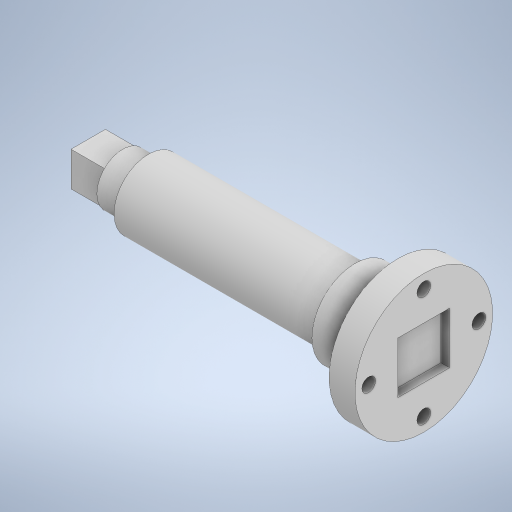
# Autodesk Inventor part: DRIVE SHAFT
Saved by Autodesk Inventor 2023 (Build 270158030, 158C)
## iProperties
Created: 2022-11-22
Part Number: DRIVE SHAFT
Material: Generic
Document SubType Name: Modeling
Designer: Imogen Heard
Density: 1 g/cm^3
Appearance: Default
Author: Imogen Heard
Autodesk Inventor part; units mm, degrees
ref_plane "YZ Plane" through (0, 0, 0) normal (1, 0, 0) x (0, 1, 0)
ref_plane "XZ Plane" through (0, 0, 0) normal (0, 1, 0) x (-1, 0, 0)
ref_plane "XY Plane" through (0, 0, 0) normal (0, 0, 1) x (1, 0, 0)
sketch "Sketch1" plane through (0, 0, 0) normal (1, 0, 0) x (0, 1, 0)
  circle A0 centre (0, 0) radius 40
  dimension "d0" = 80
  constraints: 1 centre point, 1 coincident
  measures "d0" diameter of A0
extrude "Extrusion1" add sketch "Sketch1" along normal blind 15
sketch "Sketch2" plane through (0, 0, 0) normal (-1, 0, 0) x (0, 0, 1)
  circle A0 centre (0, 0) radius 25
  circle A1 centre (0, 0) radius 40 projected
  dimension "d3" = 50
  constraints: 1 centre point, 1 concentric
  measures "d3" diameter of A0
extrude "Extrusion2" add sketch "Sketch2" along normal blind 25 contours A0
sketch "Sketch3" plane through (-25, 0, 0) normal (-1, 0, 0) x (0, 0, 1)
  circle A0 centre (0, 0) radius 20
  circle A1 centre (0, 0) radius 25 projected
  dimension "d6" = 40
  constraints: 1 centre point, 1 concentric
  measures "d6" diameter of A0
extrude "Extrusion3" add sketch "Sketch3" along normal blind 120 contours A0
sketch "Sketch4" plane through (-145, 0, 0) normal (-1, 0, 0) x (0, 0, 1)
  circle A0 centre (0, 0) radius 15
  circle A1 centre (0, 0) radius 20 projected
  dimension "d9" = 30
  constraints: 1 centre point, 1 concentric
  measures "d9" diameter of A0
extrude "Extrusion4" add sketch "Sketch4" along normal blind 15 contours A0
sketch "Sketch5" plane through (-160, 0, 0) normal (-1, 0, 0) x (0, 0, 1)
  line L0 (-10, 10) -> (10, 10)
  line L1 (10, 10) -> (10, -10)
  line L2 (10, -10) -> (-10, -10)
  line L3 (-10, -10) -> (-10, 10)
  point P0 (0, 0)
  dimension "d12" = 20
  dimension "d13" = 20
  dimension "d14" = 10
  dimension "d15" = 10
  constraints: 8 end point, 2 parallel, 1 horizontal, 1 perpendicular
  measures "d12" distance between parallel lines of L2 L0
  measures "d13" distance between parallel lines of L1 L3
  measures "d14" distance from line of point (0, 0) L3
  measures "d15" distance from line of point (0, 0) L0
extrude "Extrusion5" add sketch "Sketch5" along normal blind 20
sketch "Sketch6" plane through (15, 0, 0) normal (1, 0, 0) x (0, 0, -1)
  line L0 (-15, 15) -> (15, 15)
  line L1 (15, 15) -> (15, -15)
  line L2 (15, -15) -> (-15, -15)
  line L3 (-15, -15) -> (-15, 15)
  point P0 (0, 0)
  point P1 (-15, 0)
  point P2 (0, 15)
  dimension "d18" = 30
  dimension "d19" = 30
  dimension "d20" = 15
  dimension "d21" = 15
  constraints: 8 end point, 2 midpoint, 2 parallel, 1 horizontal, 1 perpendicular
  measures "d18" distance between parallel lines of L2 L0
  measures "d19" distance between parallel lines of L1 L3
  measures "d20" distance of point (0, 0) point (-15, 0)
  measures "d21" distance of point (0, 0) point (0, 15)
extrude "Extrusion6" cut sketch "Sketch6" against normal blind 5
sketch "Sketch7" plane through (15, 0, 0) normal (1, 0, 0) x (0, 0, -1)
  circle A0 centre (0, 32) radius 4
  circle A1 centre (32, 0) radius 4
  circle A2 centre (-32, 0) radius 4
  circle A3 centre (0, -32) radius 4
  circle A4 centre (0, 0) radius 32 construction
  circle A5 centre (0, 0) radius 40 projected
  dimension "d24" = 64
  dimension "d25" = 8
  constraints: 5 centre point, 4 point on circle, 3 equal radius, 2 horizontal alignment, 2 vertical alignment, 1 concentric
  measures "d24" diameter of A4
  measures "d25" diameter of A0
extrude "Extrusion7" cut sketch "Sketch7" against normal through all contours A0 | A1 | A2 | A3
body "Solid1"
